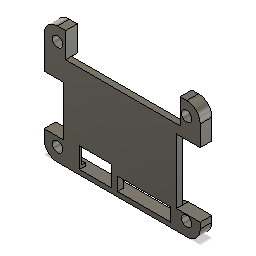
Icebreaker Case Top (Autodesk Fusion 360 design; units mm, degrees)
Autodesk Fusion 360 part; units mm, degrees
sketch "Sketch1" plane through (0, 0, 0) normal (0, 0, 1) x (1, 0, 0)
  line L0 (0, 0) -> (53.2, 0)
  line L1 (53.2, 0) -> (53.2, 40.2)
  line L2 (53.2, 40.2) -> (0, 40.2)
  line L3 (0, 40.2) -> (0, 0)
  circle A0 centre (4.6, 4.6) radius 1.75
  circle A1 centre (4.6, 35.6) radius 1.75
  circle A2 centre (48.6, 35.6) radius 1.75
  circle A3 centre (48.6, 4.6) radius 1.75
  dimension "d1" = 53.2
  dimension "d2" = 40.2
  dimension "d3" = 4.6
  dimension "d4" = 4.6
  dimension "d5" = 4.6
  dimension "d6" = 4.6
  dimension "d7" = 4.6
  dimension "d8" = 4.6
  dimension "d9" = 4.6
  dimension "d10" = 4.6
  dimension "d11" = 3.5
  dimension "d12" = 3.5
  dimension "d13" = 3.5
  dimension "d14" = 3.5
  measures "d1" distance of L0.start
  measures "d2" distance of L0.start
  measures "d3" distance of L3
  measures "d5" distance of L2
  measures "d6" distance of L3
  measures "d10" distance of L2 L0.start
  measures "d11" diameter of A1
  measures "d12" diameter of A0
  measures "d13" diameter of A3
  measures "d14" diameter of A2
extrude "Extrude1" add sketch "Sketch1" along normal blind 4
fillet "Fillet1" radius 4.6 4 edges at (0, 40.2, 2) (0, 0, 2) (53.2, 0, 2) (53.2, 40.2, 2)
sketch "Sketch2" plane through (0, 0, 0) normal (0, 0, -1) x (-1, 0, 0)
  arc A0 (-48.6, 40.2) -> (-53.2, 35.6) centre (-48.6, 35.6) ccw
  line L0 (-53.2, 35.6) -> (-53.2, 4.6)
  arc A1 (-53.2, 4.6) -> (-48.6, 0) centre (-48.6, 4.6) ccw
  line L1 (-48.6, 0) -> (-4.6, 0)
  arc A2 (-4.6, 0) -> (0, 4.6) centre (-4.6, 4.6) ccw
  line L2 (0, 4.6) -> (0, 35.6)
  arc A3 (0, 35.6) -> (-4.6, 40.2) centre (-4.6, 35.6) ccw
  line L3 (-4.6, 40.2) -> (-48.6, 40.2)
  circle A4 centre (-48.6, 4.6) radius 1.75
  circle A5 centre (-48.6, 35.6) radius 1.75
  circle A6 centre (-4.6, 4.6) radius 1.75
  circle A7 centre (-4.6, 35.6) radius 1.75
  line L4 (-51.6, 35.6) -> (-51.6, 4.6)
  arc A8 (-51.6, 4.6) -> (-48.6, 1.6) centre (-48.6, 4.6) ccw
  line L5 (-48.6, 1.6) -> (-4.6, 1.6)
  arc A9 (-4.6, 1.6) -> (-1.6, 4.6) centre (-4.6, 4.6) ccw
  line L6 (-1.6, 4.6) -> (-1.6, 35.6)
  arc A10 (-1.6, 35.6) -> (-4.6, 38.6) centre (-4.6, 35.6) ccw
  line L7 (-4.6, 38.6) -> (-48.6, 38.6)
  arc A11 (-48.6, 38.6) -> (-51.6, 35.6) centre (-48.6, 35.6) ccw
  dimension "d18" = 1.6
  measures "d18" distance of L0
extrude "Extrude2" cut sketch "Sketch2" against normal blind 2 contours L4 A8 L5 A9 L6 A10 L7 A11
sketch "Sketch3" plane through (0, 0, 0) normal (0, 0, -1) x (-1, 0, 0)
  line L0 (-51.6, 4.6) -> (-51.6, 35.6)
  arc A0 (-48.6, 38.6) -> (-51.6, 35.6) centre (-48.6, 35.6) ccw
  line L1 (-48.6, 38.6) -> (-4.6, 38.6)
  arc A1 (-1.6, 35.6) -> (-4.6, 38.6) centre (-4.6, 35.6) ccw
  line L2 (-1.6, 35.6) -> (-1.6, 4.6)
  arc A2 (-4.6, 1.6) -> (-1.6, 4.6) centre (-4.6, 4.6) ccw
  line L3 (-4.6, 1.6) -> (-48.6, 1.6)
  arc A3 (-51.6, 4.6) -> (-48.6, 1.6) centre (-48.6, 4.6) ccw
  arc A4 (-48.6, 40.2) -> (-53.2, 35.6) centre (-48.6, 35.6) ccw
  line L4 (-53.2, 35.6) -> (-53.2, 4.6)
  arc A5 (-53.2, 4.6) -> (-48.6, 0) centre (-48.6, 4.6) ccw
  line L5 (-48.6, 0) -> (-4.6, 0)
  arc A6 (-4.6, 0) -> (0, 4.6) centre (-4.6, 4.6) ccw
  line L6 (0, 4.6) -> (0, 35.6)
  arc A7 (0, 35.6) -> (-4.6, 40.2) centre (-4.6, 35.6) ccw
  line L7 (-4.6, 40.2) -> (-48.6, 40.2)
  line L8 (0, 24.6) -> (-1.6, 24.6)
  line L9 (0, 7.6) -> (-1.6, 7.6)
  line L10 (-53.2, 28.6) -> (-51.6, 28.6)
  line L11 (-53.2, 6.6) -> (-51.6, 6.6)
  line L12 (-46.35, 40.2) -> (-46.35, 38.6)
  line L13 (-7.35, 40.2) -> (-7.35, 38.6)
  dimension "d21" = 17
  dimension "d22" = 11
  dimension "d25" = 5
  dimension "d26" = 10
  dimension "d27" = 5.75
  dimension "d73" = 39
  measures "d21" distance of L8 L9
  measures "d22" distance of L8
  measures "d25" distance of L3 L11
  measures "d26" distance of L1 L10
  measures "d27" distance of L2 L13
  measures "d73" distance of L12 L13
extrude "Extrude3" cut sketch "Sketch3" against normal blind 2 contours L0 L4 L10 L11 | L2 L6 L8 L9 | L1 L7 L12 L13
sketch "Sketch4" plane through (0, 0, 2) normal (0, 0, -1) x (-1, 0, 0)
  circle A0 centre (-48.6, 4.6) radius 1.75
  circle A1 centre (-4.6, 35.6) radius 1.75
  circle A2 centre (-4.6, 4.6) radius 1.75
  circle A3 centre (-48.6, 35.6) radius 1.75
  line L0 (-53.2, 28.6) -> (-53.2, 6.6)
  line L1 (0, 7.6) -> (0, 24.6)
  line L2 (-7.35, 40.2) -> (-46.35, 40.2)
  arc A4 (-48.6, 38.6) -> (-51.6, 35.6) centre (-48.6, 35.6) ccw
  line L3 (-51.6, 35.6) -> (-51.6, 28.6)
  line L4 (-51.6, 28.6) -> (-53.2, 28.6)
  line L5 (-53.2, 6.6) -> (-51.6, 6.6)
  line L6 (-51.6, 6.6) -> (-51.6, 4.6)
  arc A5 (-51.6, 4.6) -> (-48.6, 1.6) centre (-48.6, 4.6) ccw
  line L7 (-48.6, 1.6) -> (-4.6, 1.6)
  arc A6 (-4.6, 1.6) -> (-1.6, 4.6) centre (-4.6, 4.6) ccw
  line L8 (-1.6, 4.6) -> (-1.6, 7.6)
  line L9 (-1.6, 7.6) -> (0, 7.6)
  line L10 (0, 24.6) -> (-1.6, 24.6)
  line L11 (-1.6, 24.6) -> (-1.6, 35.6)
  arc A7 (-1.6, 35.6) -> (-4.6, 38.6) centre (-4.6, 35.6) ccw
  line L12 (-4.6, 38.6) -> (-7.35, 38.6)
  line L13 (-7.35, 38.6) -> (-7.35, 40.2)
  line L14 (-46.35, 40.2) -> (-46.35, 38.6)
  line L15 (-46.35, 38.6) -> (-48.6, 38.6)
  line L16 (-51.6, 28.6) -> (-45.1, 28.6)
  line L17 (-45.1, 28.6) -> (-45.1, 6.6)
  line L18 (-45.1, 6.6) -> (-51.6, 6.6)
  line L19 (-7.35, 38.6) -> (-7.35, 31.6)
  line L20 (-7.35, 31.6) -> (-46.35, 31.6)
  line L21 (-46.35, 31.6) -> (-46.35, 38.6)
  line L22 (-1.6, 24.6) -> (-6.6, 24.6)
  line L23 (-6.6, 24.6) -> (-6.6, 7.6)
  line L24 (-6.6, 7.6) -> (-1.6, 7.6)
  line L25 (-12.1, 1.6) -> (-12.1, 8.6)
  line L26 (-12.1, 8.6) -> (-23.1, 8.6)
  line L27 (-23.1, 8.6) -> (-23.1, 1.6)
  line L28 (-25.1, 1.6) -> (-25.1, 6.1)
  line L29 (-25.1, 6.1) -> (-43.1, 6.1)
  line L30 (-43.1, 6.1) -> (-43.1, 1.6)
  dimension "d74" = 6.5
  dimension "d75" = 7
  dimension "d76" = 5
  dimension "d77" = 10.5
  dimension "d78" = 11
  dimension "d79" = 7
  dimension "d80" = 4.5
  dimension "d81" = 23.5
  dimension "d82" = 18
  measures "d74" distance of L3 L17
  measures "d75" distance of L12 L20
  measures "d76" distance of L11 L23
  measures "d77" distance of L8 L25
  measures "d79" distance of L7 L26
  measures "d80" distance of L7 L29
  measures "d81" distance of L8 L28
extrude "Extrude4" cut sketch "Sketch4" against normal blind 2 contours L0 L4 L5 L16 L17 L18 | L2 L13 L14 L19 L20 L21 | L7 L28 L29 L30 | L7 L25 L26 L27 | L1 L9 L10 L22 L23 L24
sketch "Sketch5" plane through (0, 0, 2) normal (0, 0, -1) x (-1, 0, 0)
  line L0 (-51.6, 35.6) -> (-51.6, 28.6)
  line L1 (-48.6, 1.6) -> (-43.1, 1.6)
  line L2 (-1.6, 7.6) -> (-6.6, 7.6)
  line L3 (-6.6, 24.6) -> (-1.6, 24.6)
  line L4 (-7.35, 38.6) -> (-7.35, 31.6)
  line L5 (-4.6, 38.6) -> (-7.35, 38.6)
  line L6 (-46.35, 31.6) -> (-46.35, 38.6)
  line L7 (-51.6, 28.6) -> (-45.1, 28.6)
  line L8 (-45.1, 6.6) -> (-51.6, 6.6)
  circle A0 centre (-48.6, 35.6) radius 1.75
  circle A1 centre (-4.6, 4.6) radius 1.75
  circle A2 centre (-4.6, 35.6) radius 1.75
  circle A3 centre (-48.6, 4.6) radius 1.75
  line L9 (-12.6, 8.6) -> (-6.6, 8.6)
  line L10 (-6.6, 8.6) -> (-6.6, 2.6)
  line L11 (-6.6, 2.6) -> (-12.6, 2.6)
  line L12 (-12.6, 2.6) -> (-12.6, 8.6)
  arc A4 (-4.6, 1.6) -> (-1.6, 4.6) centre (-4.6, 4.6) ccw
  line L13 (-1.6, 4.6) -> (-1.6, 7.6)
  line L14 (-1.6, 24.6) -> (-1.6, 35.6)
  arc A5 (-1.6, 35.6) -> (-4.6, 38.6) centre (-4.6, 35.6) ccw
  line L15 (-46.35, 38.6) -> (-48.6, 38.6)
  arc A6 (-48.6, 38.6) -> (-51.6, 35.6) centre (-48.6, 35.6) ccw
  line L16 (-51.6, 6.6) -> (-51.6, 4.6)
  arc A7 (-51.6, 4.6) -> (-48.6, 1.6) centre (-48.6, 4.6) ccw
  line L17 (-45.1, 28.6) -> (-45.1, 6.6)
  line L18 (-43.1, 1.6) -> (-43.1, 6.1)
  line L19 (-43.1, 6.1) -> (-25.1, 6.1)
  line L20 (-25.1, 6.1) -> (-25.1, 1.6)
  line L21 (-25.1, 1.6) -> (-23.1, 1.6)
  line L22 (-23.1, 1.6) -> (-23.1, 8.6)
  line L23 (-23.1, 8.6) -> (-12.1, 8.6)
  line L24 (-12.1, 8.6) -> (-12.1, 1.6)
  line L25 (-12.1, 1.6) -> (-4.6, 1.6)
  line L26 (-6.6, 7.6) -> (-6.6, 24.6)
  line L27 (-7.35, 31.6) -> (-46.35, 31.6)
  dimension "d49" = 6
  dimension "d51" = 6
  dimension "d83" = 1
  dimension "d84" = 5
  measures "d83" distance of L11 L25
  measures "d84" distance of L10 L13
extrude "Extrude5" cut sketch "Sketch5" against normal blind 1.3 contours L9 L10 L11 L24 L26 | L9 L11 L12 L23 L24
sketch "Sketch8" plane through (0, 0, 2) normal (0, 0, -1) x (-1, 0, 0)
  line L0 (-6.6, 24.6) -> (-1.6, 24.6)
  line L1 (-7.35, 38.6) -> (-7.35, 31.6)
  line L2 (-4.6, 38.6) -> (-7.35, 38.6)
  line L3 (-46.35, 31.6) -> (-46.35, 38.6)
  line L4 (-51.6, 28.6) -> (-45.1, 28.6)
  line L5 (-45.1, 6.6) -> (-51.6, 6.6)
  line L6 (-51.6, 35.6) -> (-51.6, 28.6)
  line L7 (-48.6, 1.6) -> (-43.1, 1.6)
  line L8 (-23.1, 8.6) -> (-6.6, 8.6)
  circle A0 centre (-48.6, 35.6) radius 1.75
  circle A1 centre (-4.6, 35.6) radius 1.75
  circle A2 centre (-48.6, 4.6) radius 1.75
  arc A3 (-1.6, 35.6) -> (-4.6, 38.6) centre (-4.6, 35.6) ccw
  line L9 (-46.35, 38.6) -> (-48.6, 38.6)
  arc A4 (-48.6, 38.6) -> (-51.6, 35.6) centre (-48.6, 35.6) ccw
  line L10 (-51.6, 6.6) -> (-51.6, 4.6)
  arc A5 (-51.6, 4.6) -> (-48.6, 1.6) centre (-48.6, 4.6) ccw
  line L11 (-6.6, 8.6) -> (-6.6, 24.6)
  line L12 (-7.35, 31.6) -> (-46.35, 31.6)
  line L13 (-45.1, 28.6) -> (-45.1, 6.6)
  line L14 (-43.1, 1.6) -> (-43.1, 6.1)
  line L15 (-43.1, 6.1) -> (-25.1, 6.1)
  line L16 (-25.1, 6.1) -> (-25.1, 1.6)
  line L17 (-25.1, 1.6) -> (-23.1, 1.6)
  line L18 (-23.1, 1.6) -> (-23.1, 8.6)
  line L19 (-1.6, 24.6) -> (-1.6, 35.6)
  line L20 (-45.1, 6.6) -> (-43.1, 6.1)
  line L21 (-7.35, 31.6) -> (-1.6, 31.6)
  line L22 (-46.35, 31.6) -> (-46.6643, 31.6)
  line L23 (-46.6643, 31.6) -> (-51.6, 31.6)
  line L24 (-6.6, 7.6) -> (-6.6, 2.6)
  line L25 (-6.6, 2.6) -> (-12.1, 2.6)
  line L26 (-12.1, 2.6) -> (-12.1, 1.6)
  line L27 (-12.1, 1.6) -> (-4.6, 1.6)
  arc A6 (-4.6, 1.6) -> (-1.6, 4.6) centre (-4.6, 4.6) ccw
  line L28 (-1.6, 4.6) -> (-1.6, 7.6)
  line L29 (-1.6, 7.6) -> (-6.6, 7.6)
  circle A7 centre (-4.6, 4.6) radius 1.75
  line L30 (-6.6, 2.6) -> (-6.6, 1.6)
extrude "Extrude8" add sketch "Sketch8" along normal blind 2 contours L1 L2 A3 L19 L21 | L3 L6 L9 A4 L22 L23 | L5 L7 L10 A5 L14 L20 | L24 L27 A6 L28 L29 L30
sketch "Sketch9" plane through (0, 0, 2) normal (0, 0, -1) x (-1, 0, 0)
  line L0 (-45.1, 6.6) -> (-43.1, 6.1)
  line L1 (-43.1, 6.1) -> (-25.1, 6.1)
  line L2 (-25.1, 6.1) -> (-25.1, 1.6)
  line L3 (-25.1, 1.6) -> (-23.1, 1.6)
  line L4 (-23.1, 1.6) -> (-23.1, 8.6)
  line L5 (-23.1, 8.6) -> (-6.6, 8.6)
  line L6 (-6.6, 8.6) -> (-6.6, 24.6)
  line L7 (-6.6, 24.6) -> (-1.6, 24.6)
  line L8 (-1.6, 24.6) -> (-1.6, 31.6)
  line L9 (-1.6, 31.6) -> (-7.35, 31.6)
  line L10 (-7.35, 31.6) -> (-46.35, 31.6)
  line L11 (-46.35, 31.6) -> (-51.6, 31.6)
  line L12 (-51.6, 31.6) -> (-51.6, 28.6)
  line L13 (-51.6, 28.6) -> (-45.1, 28.6)
  line L14 (-45.1, 28.6) -> (-45.1, 6.6)
  line L15 (-7.6, 10.6) -> (-9.6, 10.6)
  line L16 (-9.6, 10.6) -> (-9.6, 13.6)
  line L17 (-9.6, 13.6) -> (-7.6, 13.6)
  line L18 (-7.6, 13.6) -> (-7.6, 10.6)
  dimension "d85" = 2
  dimension "d86" = 1
  dimension "d87" = 3
  dimension "d88" = 2
  measures "d85" distance of L5 L15
  measures "d86" distance of L6 L18
extrude "Extrude9" cut sketch "Sketch9" against normal blind 1.5 contours L15 L16 L17 L18
equation "d1 = 50 mm + ( ( 2 * 1.6 ) * 1 mm )"
equation "d2 = 37 mm + ( ( 2 * 1.6 ) * 1 mm )"
equation "d3 = 3 mm + 1.6 mm"
equation "d4 = d3"
equation "d5 = d4"
equation "d6 = d3"
equation "d7 = d3"
equation "d8 = d7"
equation "d9 = d4"
equation "d10 = d5"
equation "d17 = 3 mm + 1.6 mm"
